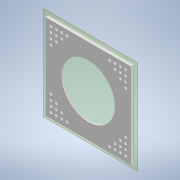
# Autodesk Inventor part: 60T-LocatorPlate
Saved by Autodesk Inventor 2020 (Build 240168000, 168)
## iProperties
Created: 2020-01-23
Part Number: 60T-LocatorPlate
Material: Generic
Document SubType Name: Modeling
Designer: srini
Density: 1 g/cm^3
Appearance: Default
Author: srini
Autodesk Inventor part; units mm, degrees
(part 1 of 2)
ref_plane "YZ Plane" through (0, 0, 0) normal (1, 0, 0) x (0, 1, 0)
ref_plane "XZ Plane" through (0, 0, 0) normal (0, 1, 0) x (-1, 0, 0)
ref_plane "XY Plane" through (0, 0, 0) normal (0, 0, 1) x (1, 0, 0)
sketch "Sketch1" plane through (0, 0, 0) normal (0, 0, 1) x (1, 0, 0)
  line L0 (-101.6, 101.6) -> (101.6, 101.6)
  line L1 (101.6, 101.6) -> (101.6, -101.6)
  line L2 (101.6, -101.6) -> (-101.6, -101.6)
  line L3 (-101.6, -101.6) -> (-101.6, 101.6)
  line L4 (-101.6, 101.6) -> (101.6, -101.6) construction
  line L5 (101.6, 101.6) -> (-101.6, -101.6) construction
  point P0 (0, 0)
  dimension "d0" = 203.2
  constraints: 12 end point, 2 midpoint, 2 parallel, 2 perpendicular, 1 horizontal
  measures "d0" distance of L0.start L0.end
extrude "Extrusion1" add sketch "Sketch1" along normal blind 3.175
ref_plane "Work Plane1" through (0, 0, -2.1465) normal (0, 0, -1) x (-1, 0, 0)
sketch "Sketch2" plane through (0, 0, -2.1465) normal (0, 0, -1) x (-1, 0, 0)
  circle A0 centre (0, 0) radius 14.3 construction
  circle A1 centre (20.6222, 11.9063) radius 2.1526 construction
  circle A2 centre (20.6222, -11.9062) radius 2.1526 construction
  circle A3 centre (0, -23.8125) radius 2.1526 construction
  circle A4 centre (-20.6222, -11.9063) radius 2.1526 construction
  circle A5 centre (-20.6222, 11.9062) radius 2.1526 construction
  circle A6 centre (0, 23.8125) radius 2.1526 construction
  arc A7 (-93.6337, -4.2799) -> (-93.5681, -5.531) centre (0, 0) ccw construction
  arc A8 (-92.0229, -3.2534) -> (-93.6337, -4.2799) centre (-90.7026, -7.1023) ccw construction
  line L0 (-92.0229, -3.2534) -> (-91.3043, -3.0069) construction
  arc A9 (-91.3043, -3.0069) -> (-89.552, -2.096) centre (-93.4636, 3.2878) ccw construction
  arc A10 (-89.552, -2.096) -> (-89.552, 2.096) centre (-91.0748, 0) ccw construction
  arc A11 (-89.552, 2.096) -> (-91.3043, 3.0069) centre (-93.4636, -3.2878) ccw construction
  line L1 (-91.3043, 3.0069) -> (-92.0229, 3.2534) construction
  arc A12 (-93.6337, 4.2799) -> (-92.0229, 3.2534) centre (-90.7026, 7.1023) ccw construction
  arc A13 (-93.5681, 5.531) -> (-93.6337, 4.2799) centre (0, 0) ccw construction
  arc A14 (-91.8588, 6.3834) -> (-93.5681, 5.531) centre (-90.9481, 2.4177) ccw construction
  line L2 (-91.8588, 6.3834) -> (-91.1184, 6.5535) construction
  arc A15 (-91.1184, 6.5535) -> (-89.2805, 7.2762) centre (-92.6079, 13.0394) ccw construction
  arc A16 (-89.2805, 7.2762) -> (-88.8423, 11.4453) centre (-90.5759, 9.5199) ccw construction
  arc A17 (-88.8423, 11.4453) -> (-90.4898, 12.5343) centre (-93.2953, 6.4998) ccw construction
  line L3 (-90.4898, 12.5343) -> (-91.1787, 12.8546) construction
  arc A18 (-92.6733, 14.0438) -> (-91.1787, 12.8546) centre (-89.4633, 16.5444) ccw construction
  arc A19 (-92.4774, 15.2812) -> (-92.6733, 14.0438) centre (0, 0) ccw construction
  arc A20 (-90.6884, 15.9503) -> (-92.4774, 15.2812) centre (-90.1972, 11.9111) ccw construction
  line L4 (-90.6884, 15.9503) -> (-89.9343, 16.042) construction
  arc A21 (-89.9343, 16.042) -> (-88.0308, 16.5687) centre (-90.7376, 22.6482) ccw construction
  arc A22 (-88.0308, 16.5687) -> (-87.1593, 20.6691) centre (-89.0846, 18.9355) ccw construction
  arc A23 (-87.1593, 20.6691) -> (-88.6839, 21.9244) centre (-92.1048, 16.2162) ccw construction
  line L5 (-88.6839, 21.9244) -> (-89.3355, 22.3149) construction
  arc A24 (-90.6977, 23.6539) -> (-89.3355, 22.3149) centre (-87.2439, 25.8052) ccw construction
  arc A25 (-90.3734, 24.864) -> (-90.6977, 23.6539) centre (0, 0) ccw construction
  arc A26 (-88.5243, 25.3425) -> (-90.3734, 24.864) centre (-88.458, 21.274) ccw construction
  line L6 (-88.5243, 25.3425) -> (-87.7647, 25.3548) construction
  arc A27 (-87.7647, 25.3548) -> (-85.8167, 25.6797) centre (-87.8731, 32.0088) ccw construction
  arc A28 (-85.8167, 25.6797) -> (-84.5213, 29.6665) centre (-86.6173, 28.1437) ccw construction
  arc A29 (-84.5213, 29.6665) -> (-85.9064, 31.0743) centre (-89.9051, 25.7549) ccw construction
  line L7 (-85.9064, 31.0743) -> (-86.5136, 31.5308) construction
  arc A30 (-87.7283, 33.0048) -> (-86.5136, 31.5308) centre (-84.0686, 34.7833) ccw construction
  arc A31 (-87.2794, 34.1744) -> (-87.7283, 33.0048) centre (0, 0) ccw construction
  arc A32 (-85.3904, 34.4569) -> (-87.2794, 34.1744) centre (-85.7497, 30.4038) ccw construction
  line L8 (-85.3904, 34.4569) -> (-84.6337, 34.3899) construction
  arc A33 (-84.6337, 34.3899) -> (-82.6623, 34.5093) centre (-84.0459, 41.0187) ccw construction
  arc A34 (-82.6623, 34.5093) -> (-80.9573, 38.3389) centre (-83.201, 37.0435) ccw construction
  arc A35 (-80.9573, 38.3389) -> (-82.1876, 39.8837) centre (-86.7205, 35.0115) ccw construction
  line L9 (-82.1876, 39.8837) -> (-82.7438, 40.4012) construction
  arc A36 (-83.7978, 41.9941) -> (-82.7438, 40.4012) centre (-79.9722, 43.3803) ccw construction
  arc A37 (-83.2291, 43.1103) -> (-83.7978, 41.9941) centre (0, 0) ccw construction
  arc A38 (-81.3208, 43.1939) -> (-83.2291, 43.1103) centre (-82.1019, 39.2006) ccw construction
  line L10 (-81.3208, 43.1939) -> (-80.5753, 43.0481) construction
  arc A39 (-80.5753, 43.0481) -> (-78.6023, 42.9608) centre (-79.2979, 49.5791) ccw construction
  arc A40 (-78.6023, 42.9608) -> (-76.5063, 46.5912) centre (-78.8731, 45.5374) ccw construction
  arc A41 (-76.5063, 46.5912) -> (-77.5684, 48.2562) centre (-82.5858, 43.8844) ccw construction
  line L11 (-77.5684, 48.2562) -> (-78.0675, 48.829) construction
  arc A42 (-78.9492, 50.5233) -> (-78.0675, 48.829) centre (-74.9996, 51.502) ccw construction
  arc A43 (-78.2669, 51.574) -> (-78.9492, 50.5233) centre (0, 0) ccw construction
  arc A44 (-76.3604, 51.4576) -> (-78.2669, 51.574) centre (-77.5546, 47.5678) ccw construction
  line L12 (-76.3604, 51.4576) -> (-75.6342, 51.2347) construction
  arc A45 (-75.6342, 51.2347) -> (-73.6811, 50.9416) centre (-73.6811, 57.5964) ccw construction
  arc A46 (-73.6811, 50.9416) -> (-71.2171, 54.333) centre (-73.6811, 53.5324) ccw construction
  arc A47 (-71.2171, 54.333) -> (-72.0993, 56.1) centre (-77.5462, 52.2766) ccw construction
  line L13 (-72.0993, 56.1) -> (-72.5358, 56.7217) construction
  arc A48 (-73.2356, 58.499) -> (-72.5358, 56.7217) centre (-69.2054, 59.0595) ccw construction
  arc A49 (-72.4472, 59.4726) -> (-73.2356, 58.499) centre (0, 0) ccw construction
  arc A50 (-70.5633, 59.1576) -> (-72.4472, 59.4726) centre (-72.1575, 55.4139) ccw construction
  line L14 (-70.5633, 59.1576) -> (-69.8643, 58.8599) construction
  arc A51 (-69.8643, 58.8599) -> (-67.9526, 58.3643) centre (-67.257, 64.9827) ccw construction
  arc A52 (-67.9526, 58.3643) -> (-65.1476, 61.4796) centre (-67.6818, 60.9409) ccw construction
  arc A53 (-65.1476, 61.4796) -> (-65.8403, 63.3291) centre (-71.657, 60.096) ccw construction
  line L15 (-65.8403, 63.3291) -> (-66.2094, 63.9931) construction
  arc A54 (-66.7196, 65.8337) -> (-66.2094, 63.9931) centre (-62.6528, 65.9699) ccw construction
  arc A55 (-65.8337, 66.7196) -> (-66.7196, 65.8337) centre (0, 0) ccw construction
  arc A56 (-63.9931, 66.2094) -> (-65.8337, 66.7196) centre (-65.9699, 62.6528) ccw construction
  line L16 (-63.9931, 66.2094) -> (-63.3291, 65.8403) construction
  arc A57 (-63.3291, 65.8403) -> (-61.4796, 65.1476) centre (-60.096, 71.657) ccw construction
  arc A58 (-61.4796, 65.1476) -> (-58.3643, 67.9526) centre (-60.941, 67.6818) ccw construction
  arc A59 (-58.3643, 67.9526) -> (-58.8599, 69.8643) centre (-64.9827, 67.257) ccw construction
  line L17 (-58.8599, 69.8643) -> (-59.1576, 70.5633) construction
  arc A60 (-59.4726, 72.4472) -> (-59.1576, 70.5633) centre (-55.4139, 72.1575) ccw construction
  arc A61 (-58.499, 73.2356) -> (-59.4726, 72.4472) centre (0, 0) ccw construction
  arc A62 (-56.7217, 72.5358) -> (-58.499, 73.2356) centre (-59.0595, 69.2053) ccw construction
  line L18 (-56.7217, 72.5358) -> (-56.1, 72.0993) construction
  arc A63 (-56.1, 72.0993) -> (-54.333, 71.2171) centre (-52.2766, 77.5462) ccw construction
  arc A64 (-54.333, 71.2171) -> (-50.9416, 73.6811) centre (-53.5324, 73.6811) ccw construction
  arc A65 (-50.9416, 73.6811) -> (-51.2347, 75.6341) centre (-57.5964, 73.6811) ccw construction
  line L19 (-51.2347, 75.6341) -> (-51.4576, 76.3604) construction
  arc A66 (-51.574, 78.2669) -> (-51.4576, 76.3604) centre (-47.5678, 77.5545) ccw construction
  arc A67 (-50.5233, 78.9492) -> (-51.574, 78.2669) centre (0, 0) ccw construction
  arc A68 (-48.829, 78.0674) -> (-50.5233, 78.9492) centre (-51.502, 74.9996) ccw construction
  line L20 (-48.829, 78.0674) -> (-48.2562, 77.5684) construction
  arc A69 (-48.2562, 77.5684) -> (-46.5912, 76.5063) centre (-43.8844, 82.5858) ccw construction
  arc A70 (-46.5912, 76.5063) -> (-42.9608, 78.6023) centre (-45.5374, 78.8731) ccw construction
  arc A71 (-42.9608, 78.6023) -> (-43.0481, 80.5753) centre (-49.5792, 79.2979) ccw construction
  line L21 (-43.0481, 80.5753) -> (-43.1939, 81.3208) construction
  arc A72 (-43.1103, 83.2291) -> (-43.1939, 81.3208) centre (-39.2006, 82.1019) ccw construction
  arc A73 (-41.9941, 83.7978) -> (-43.1103, 83.2291) centre (0, 0) ccw construction
  arc A74 (-40.4012, 82.7438) -> (-41.9941, 83.7978) centre (-43.3803, 79.9722) ccw construction
  line L22 (-40.4012, 82.7438) -> (-39.8838, 82.1876) construction
  arc A75 (-39.8838, 82.1876) -> (-38.3389, 80.9573) centre (-35.0115, 86.7205) ccw construction
  arc A76 (-38.3389, 80.9573) -> (-34.5093, 82.6623) centre (-37.0435, 83.201) ccw construction
  arc A77 (-34.5093, 82.6623) -> (-34.3899, 84.6336) centre (-41.0187, 84.0459) ccw construction
  line L23 (-34.3899, 84.6336) -> (-34.457, 85.3904) construction
  arc A78 (-34.1744, 87.2794) -> (-34.457, 85.3904) centre (-30.4038, 85.7497) ccw construction
  arc A79 (-33.0048, 87.7283) -> (-34.1744, 87.2794) centre (0, 0) ccw construction
  arc A80 (-31.5308, 86.5136) -> (-33.0048, 87.7283) centre (-34.7833, 84.0686) ccw construction
  line L24 (-31.5308, 86.5136) -> (-31.0743, 85.9064) construction
  arc A81 (-31.0743, 85.9064) -> (-29.6665, 84.5213) centre (-25.7549, 89.9051) ccw construction
  arc A82 (-29.6665, 84.5213) -> (-25.6797, 85.8167) centre (-28.1437, 86.6173) ccw construction
  arc A83 (-25.6797, 85.8167) -> (-25.3548, 87.7647) centre (-32.0088, 87.8731) ccw construction
  line L25 (-25.3548, 87.7647) -> (-25.3425, 88.5243) construction
  arc A84 (-24.864, 90.3734) -> (-25.3425, 88.5243) centre (-21.274, 88.458) ccw construction
  arc A85 (-23.6539, 90.6977) -> (-24.864, 90.3734) centre (0, 0) ccw construction
  arc A86 (-22.3149, 89.3355) -> (-23.6539, 90.6977) centre (-25.8052, 87.2439) ccw construction
  line L26 (-22.3149, 89.3355) -> (-21.9244, 88.6839) construction
  arc A87 (-21.9244, 88.6839) -> (-20.6691, 87.1593) centre (-16.2162, 92.1048) ccw construction
  arc A88 (-20.6691, 87.1593) -> (-16.5687, 88.0308) centre (-18.9355, 89.0846) ccw construction
  arc A89 (-16.5687, 88.0308) -> (-16.042, 89.9343) centre (-22.6482, 90.7376) ccw construction
  line L27 (-16.042, 89.9343) -> (-15.9503, 90.6884) construction
  arc A90 (-15.2812, 92.4774) -> (-15.9503, 90.6884) centre (-11.9111, 90.1972) ccw construction
  arc A91 (-14.0438, 92.6733) -> (-15.2812, 92.4774) centre (0, 0) ccw construction
  arc A92 (-12.8546, 91.1787) -> (-14.0438, 92.6733) centre (-16.5444, 89.4633) ccw construction
  line L28 (-12.8546, 91.1787) -> (-12.5343, 90.4898) construction
  arc A93 (-12.5343, 90.4898) -> (-11.4453, 88.8423) centre (-6.4998, 93.2952) ccw construction
  arc A94 (-11.4453, 88.8423) -> (-7.2762, 89.2805) centre (-9.5199, 90.5759) ccw construction
  arc A95 (-7.2762, 89.2805) -> (-6.5535, 91.1184) centre (-13.0394, 92.6079) ccw construction
  line L29 (-6.5535, 91.1184) -> (-6.3834, 91.8588) construction
  arc A96 (-5.531, 93.5681) -> (-6.3834, 91.8588) centre (-2.4177, 90.9481) ccw construction
  arc A97 (-4.2799, 93.6336) -> (-5.531, 93.5681) centre (0, 0) ccw construction
  arc A98 (-3.2534, 92.0229) -> (-4.2799, 93.6336) centre (-7.1023, 90.7026) ccw construction
  line L30 (-3.2534, 92.0229) -> (-3.0069, 91.3043) construction
  arc A99 (-3.0069, 91.3043) -> (-2.096, 89.552) centre (3.2878, 93.4636) ccw construction
  arc A100 (-2.096, 89.552) -> (2.096, 89.552) centre (0, 91.0748) ccw construction
  arc A101 (2.096, 89.552) -> (3.0069, 91.3043) centre (-3.2878, 93.4636) ccw construction
  line L31 (3.0069, 91.3043) -> (3.2534, 92.0229) construction
  arc A102 (4.2799, 93.6336) -> (3.2534, 92.0229) centre (7.1022, 90.7026) ccw construction
  arc A103 (5.5309, 93.5681) -> (4.2799, 93.6336) centre (0, 0) ccw construction
  arc A104 (6.3834, 91.8588) -> (5.5309, 93.5681) centre (2.4177, 90.9481) ccw construction
  line L32 (6.3834, 91.8588) -> (6.5535, 91.1184) construction
  arc A105 (6.5535, 91.1184) -> (7.2762, 89.2805) centre (13.0394, 92.6079) ccw construction
  arc A106 (7.2762, 89.2805) -> (11.4452, 88.8423) centre (9.5199, 90.5759) ccw construction
  arc A107 (11.4452, 88.8423) -> (12.5343, 90.4898) centre (6.4998, 93.2952) ccw construction
  line L33 (12.5343, 90.4898) -> (12.8546, 91.1787) construction
  arc A108 (14.0438, 92.6733) -> (12.8546, 91.1787) centre (16.5443, 89.4633) ccw construction
  arc A109 (15.2812, 92.4774) -> (14.0438, 92.6733) centre (0, 0) ccw construction
  arc A110 (15.9503, 90.6884) -> (15.2812, 92.4774) centre (11.9111, 90.1972) ccw construction
  line L34 (15.9503, 90.6884) -> (16.042, 89.9343) construction
  arc A111 (16.042, 89.9343) -> (16.5687, 88.0308) centre (22.6482, 90.7376) ccw construction
  arc A112 (16.5687, 88.0308) -> (20.6691, 87.1593) centre (18.9355, 89.0846) ccw construction
  arc A113 (20.6691, 87.1593) -> (21.9244, 88.6839) centre (16.2162, 92.1048) ccw construction
  line L35 (21.9244, 88.6839) -> (22.3149, 89.3355) construction
  arc A114 (23.6539, 90.6977) -> (22.3149, 89.3355) centre (25.8052, 87.2439) ccw construction
  arc A115 (24.864, 90.3734) -> (23.6539, 90.6977) centre (0, 0) ccw construction
  arc A116 (25.3425, 88.5243) -> (24.864, 90.3734) centre (21.274, 88.458) ccw construction
  line L36 (25.3425, 88.5243) -> (25.3548, 87.7647) construction
  arc A117 (25.3548, 87.7647) -> (25.6797, 85.8167) centre (32.0088, 87.8731) ccw construction
  arc A118 (25.6797, 85.8167) -> (29.6665, 84.5213) centre (28.1437, 86.6173) ccw construction
  arc A119 (29.6665, 84.5213) -> (31.0743, 85.9064) centre (25.7549, 89.9051) ccw construction
  line L37 (31.0743, 85.9064) -> (31.5308, 86.5136) construction
  arc A120 (33.0048, 87.7283) -> (31.5308, 86.5136) centre (34.7833, 84.0686) ccw construction
  arc A121 (34.1744, 87.2794) -> (33.0048, 87.7283) centre (0, 0) ccw construction
  arc A122 (34.4569, 85.3903) -> (34.1744, 87.2794) centre (30.4038, 85.7497) ccw construction
  line L38 (34.4569, 85.3903) -> (34.3899, 84.6337) construction
  arc A123 (34.3899, 84.6337) -> (34.5093, 82.6623) centre (41.0187, 84.0459) ccw construction
  arc A124 (34.5093, 82.6623) -> (38.3389, 80.9573) centre (37.0435, 83.201) ccw construction
  arc A125 (38.3389, 80.9573) -> (39.8837, 82.1876) centre (35.0115, 86.7205) ccw construction
  line L39 (39.8837, 82.1876) -> (40.4012, 82.7438) construction
  arc A126 (41.9941, 83.7978) -> (40.4012, 82.7438) centre (43.3803, 79.9722) ccw construction
  arc A127 (43.1103, 83.2291) -> (41.9941, 83.7978) centre (0, 0) ccw construction
  arc A128 (43.1939, 81.3208) -> (43.1103, 83.2291) centre (39.2006, 82.1019) ccw construction
  line L40 (43.1939, 81.3208) -> (43.0481, 80.5753) construction
  arc A129 (43.0481, 80.5753) -> (42.9608, 78.6023) centre (49.5791, 79.2979) ccw construction
  arc A130 (42.9608, 78.6023) -> (46.5912, 76.5063) centre (45.5374, 78.8731) ccw construction
  arc A131 (46.5912, 76.5063) -> (48.2562, 77.5684) centre (43.8844, 82.5858) ccw construction
  line L41 (48.2562, 77.5684) -> (48.829, 78.0674) construction
  arc A132 (50.5233, 78.9492) -> (48.829, 78.0674) centre (51.502, 74.9996) ccw construction
  arc A133 (51.574, 78.2669) -> (50.5233, 78.9492) centre (0, 0) ccw construction
  arc A134 (51.4576, 76.3604) -> (51.574, 78.2669) centre (47.5678, 77.5545) ccw construction
  line L42 (51.4576, 76.3604) -> (51.2347, 75.6342) construction
  arc A135 (51.2347, 75.6342) -> (50.9416, 73.6811) centre (57.5964, 73.6811) ccw construction
  arc A136 (50.9416, 73.6811) -> (54.333, 71.2171) centre (53.5324, 73.6811) ccw construction
  arc A137 (54.333, 71.2171) -> (56.1, 72.0993) centre (52.2766, 77.5462) ccw construction
  line L43 (56.1, 72.0993) -> (56.7217, 72.5358) construction
  arc A138 (58.499, 73.2356) -> (56.7217, 72.5358) centre (59.0595, 69.2053) ccw construction
  arc A139 (59.4726, 72.4472) -> (58.499, 73.2356) centre (0, 0) ccw construction
  arc A140 (59.1576, 70.5633) -> (59.4726, 72.4472) centre (55.4139, 72.1575) ccw construction
  line L44 (59.1576, 70.5633) -> (58.8599, 69.8643) construction
  arc A141 (58.8599, 69.8643) -> (58.3643, 67.9526) centre (64.9827, 67.257) ccw construction
  arc A142 (58.3643, 67.9526) -> (61.4796, 65.1476) centre (60.9409, 67.6818) ccw construction
  arc A143 (61.4796, 65.1476) -> (63.3291, 65.8403) centre (60.096, 71.657) ccw construction
  line L45 (63.3291, 65.8403) -> (63.9931, 66.2094) construction
  arc A144 (65.8337, 66.7196) -> (63.9931, 66.2094) centre (65.9699, 62.6528) ccw construction
  arc A145 (66.7196, 65.8337) -> (65.8337, 66.7196) centre (0, 0) ccw construction
  arc A146 (66.2094, 63.9931) -> (66.7196, 65.8337) centre (62.6528, 65.9699) ccw construction
  line L46 (66.2094, 63.9931) -> (65.8403, 63.3291) construction
  arc A147 (65.8403, 63.3291) -> (65.1476, 61.4796) centre (71.657, 60.096) ccw construction
  arc A148 (65.1476, 61.4796) -> (67.9526, 58.3643) centre (67.6818, 60.9409) ccw construction
  arc A149 (67.9526, 58.3643) -> (69.8643, 58.8599) centre (67.257, 64.9827) ccw construction
  line L47 (69.8643, 58.8599) -> (70.5633, 59.1576) construction
  arc A150 (72.4472, 59.4726) -> (70.5633, 59.1576) centre (72.1575, 55.4139) ccw construction
  arc A151 (73.2356, 58.499) -> (72.4472, 59.4726) centre (0, 0) ccw construction
  arc A152 (72.5358, 56.7217) -> (73.2356, 58.499) centre (69.2053, 59.0595) ccw construction
  line L48 (72.5358, 56.7217) -> (72.0993, 56.1) construction
  arc A153 (72.0993, 56.1) -> (71.2171, 54.333) centre (77.5462, 52.2766) ccw construction
  arc A154 (71.2171, 54.333) -> (73.6811, 50.9416) centre (73.6811, 53.5324) ccw construction
  arc A155 (73.6811, 50.9416) -> (75.6341, 51.2347) centre (73.6811, 57.5964) ccw construction
  line L49 (75.6341, 51.2347) -> (76.3604, 51.4576) construction
  arc A156 (78.2669, 51.574) -> (76.3604, 51.4576) centre (77.5545, 47.5678) ccw construction
  arc A157 (78.9492, 50.5233) -> (78.2669, 51.574) centre (0, 0) ccw construction
  arc A158 (78.0674, 48.829) -> (78.9492, 50.5233) centre (74.9996, 51.502) ccw construction
  line L50 (78.0674, 48.829) -> (77.5684, 48.2562) construction
  arc A159 (77.5684, 48.2562) -> (76.5063, 46.5912) centre (82.5858, 43.8844) ccw construction
  arc A160 (76.5063, 46.5912) -> (78.6023, 42.9608) centre (78.8731, 45.5374) ccw construction
  arc A161 (78.6023, 42.9608) -> (80.5753, 43.0481) centre (79.2979, 49.5791) ccw construction
  line L51 (80.5753, 43.0481) -> (81.3208, 43.1939) construction
  arc A162 (83.229, 43.1103) -> (81.3208, 43.1939) centre (82.1019, 39.2006) ccw construction
  arc A163 (83.7978, 41.9941) -> (83.229, 43.1103) centre (0, 0) ccw construction
  arc A164 (82.7438, 40.4012) -> (83.7978, 41.9941) centre (79.9722, 43.3803) ccw construction
  line L52 (82.7438, 40.4012) -> (82.1876, 39.8838) construction
  arc A165 (82.1876, 39.8838) -> (80.9573, 38.3389) centre (86.7205, 35.0115) ccw construction
  arc A166 (80.9573, 38.3389) -> (82.6623, 34.5093) centre (83.201, 37.0435) ccw construction
  arc A167 (82.6623, 34.5093) -> (84.6336, 34.3899) centre (84.0459, 41.0187) ccw construction
  line L53 (84.6336, 34.3899) -> (85.3903, 34.4569) construction
  arc A168 (87.2794, 34.1744) -> (85.3903, 34.4569) centre (85.7497, 30.4038) ccw construction
  arc A169 (87.7283, 33.0048) -> (87.2794, 34.1744) centre (0, 0) ccw construction
  arc A170 (86.5136, 31.5308) -> (87.7283, 33.0048) centre (84.0686, 34.7833) ccw construction
  line L54 (86.5136, 31.5308) -> (85.9064, 31.0743) construction
  arc A171 (85.9064, 31.0743) -> (84.5213, 29.6665) centre (89.9051, 25.7549) ccw construction
  arc A172 (84.5213, 29.6665) -> (85.8167, 25.6797) centre (86.6173, 28.1437) ccw construction
  arc A173 (85.8167, 25.6797) -> (87.7647, 25.3548) centre (87.8731, 32.0088) ccw construction
  line L55 (87.7647, 25.3548) -> (88.5243, 25.3425) construction
  arc A174 (90.3734, 24.864) -> (88.5243, 25.3425) centre (88.458, 21.274) ccw construction
  arc A175 (90.6977, 23.6539) -> (90.3734, 24.864) centre (0, 0) ccw construction
  arc A176 (89.3355, 22.3149) -> (90.6977, 23.6539) centre (87.2439, 25.8052) ccw construction
  line L56 (89.3355, 22.3149) -> (88.6839, 21.9244) construction
  arc A177 (88.6839, 21.9244) -> (87.1593, 20.6691) centre (92.1048, 16.2162) ccw construction
  arc A178 (87.1593, 20.6691) -> (88.0308, 16.5687) centre (89.0846, 18.9355) ccw construction
  arc A179 (88.0308, 16.5687) -> (89.9342, 16.042) centre (90.7376, 22.6482) ccw construction
  line L57 (89.9342, 16.042) -> (90.6884, 15.9503) construction
  arc A180 (92.4774, 15.2812) -> (90.6884, 15.9503) centre (90.1972, 11.9111) ccw construction
  arc A181 (92.6733, 14.0438) -> (92.4774, 15.2812) centre (0, 0) ccw construction
  arc A182 (91.1787, 12.8546) -> (92.6733, 14.0438) centre (89.4633, 16.5443) ccw construction
  line L58 (91.1787, 12.8546) -> (90.4898, 12.5343) construction
  arc A183 (90.4898, 12.5343) -> (88.8423, 11.4452) centre (93.2952, 6.4998) ccw construction
  arc A184 (88.8423, 11.4452) -> (89.2805, 7.2762) centre (90.5759, 9.5199) ccw construction
  arc A185 (89.2805, 7.2762) -> (91.1184, 6.5535) centre (92.6079, 13.0394) ccw construction
  line L59 (91.1184, 6.5535) -> (91.8588, 6.3834) construction
  arc A186 (93.5681, 5.5309) -> (91.8588, 6.3834) centre (90.9481, 2.4177) ccw construction
  arc A187 (93.6336, 4.2799) -> (93.5681, 5.5309) centre (0, 0) ccw construction
  arc A188 (92.0229, 3.2534) -> (93.6336, 4.2799) centre (90.7026, 7.1022) ccw construction
  line L60 (92.0229, 3.2534) -> (91.3043, 3.0069) construction
  arc A189 (91.3043, 3.0069) -> (89.552, 2.096) centre (93.4636, -3.2878) ccw construction
  arc A190 (89.552, 2.096) -> (89.552, -2.096) centre (91.0748, 0) ccw construction
  arc A191 (89.552, -2.096) -> (91.3043, -3.0069) centre (93.4636, 3.2878) ccw construction
  line L61 (91.3043, -3.0069) -> (92.0229, -3.2534) construction
  arc A192 (93.6336, -4.2799) -> (92.0229, -3.2534) centre (90.7026, -7.1023) ccw construction
  arc A193 (93.5681, -5.531) -> (93.6336, -4.2799) centre (0, 0) ccw construction
  arc A194 (91.8588, -6.3834) -> (93.5681, -5.531) centre (90.9481, -2.4177) ccw construction
  line L62 (91.8588, -6.3834) -> (91.1184, -6.5535) construction
  arc A195 (91.1184, -6.5535) -> (89.2805, -7.2762) centre (92.6079, -13.0394) ccw construction
  arc A196 (89.2805, -7.2762) -> (88.8423, -11.4453) centre (90.5759, -9.5199) ccw construction
  arc A197 (88.8423, -11.4453) -> (90.4898, -12.5343) centre (93.2952, -6.4998) ccw construction
  line L63 (90.4898, -12.5343) -> (91.1787, -12.8546) construction
  arc A198 (92.6733, -14.0438) -> (91.1787, -12.8546) centre (89.4633, -16.5444) ccw construction
  arc A199 (92.4774, -15.2812) -> (92.6733, -14.0438) centre (0, 0) ccw construction
  arc A200 (90.6884, -15.9503) -> (92.4774, -15.2812) centre (90.1972, -11.9111) ccw construction
  line L64 (90.6884, -15.9503) -> (89.9343, -16.042) construction
  arc A201 (89.9343, -16.042) -> (88.0308, -16.5687) centre (90.7376, -22.6482) ccw construction
  arc A202 (88.0308, -16.5687) -> (87.1593, -20.6691) centre (89.0846, -18.9355) ccw construction
  arc A203 (87.1593, -20.6691) -> (88.6839, -21.9244) centre (92.1048, -16.2162) ccw construction
  line L65 (88.6839, -21.9244) -> (89.3355, -22.3149) construction
  arc A204 (90.6977, -23.6539) -> (89.3355, -22.3149) centre (87.2439, -25.8052) ccw construction
  arc A205 (90.3734, -24.864) -> (90.6977, -23.6539) centre (0, 0) ccw construction
  arc A206 (88.5243, -25.3425) -> (90.3734, -24.864) centre (88.458, -21.274) ccw construction
  line L66 (88.5243, -25.3425) -> (87.7647, -25.3548) construction
  arc A207 (87.7647, -25.3548) -> (85.8167, -25.6797) centre (87.8731, -32.0088) ccw construction
  arc A208 (85.8167, -25.6797) -> (84.5213, -29.6665) centre (86.6173, -28.1437) ccw construction
  arc A209 (84.5213, -29.6665) -> (85.9064, -31.0743) centre (89.9051, -25.7549) ccw construction
  line L67 (85.9064, -31.0743) -> (86.5136, -31.5308) construction
  arc A210 (87.7283, -33.0048) -> (86.5136, -31.5308) centre (84.0686, -34.7833) ccw construction
  arc A211 (87.2794, -34.1744) -> (87.7283, -33.0048) centre (0, 0) ccw construction
  arc A212 (85.3903, -34.457) -> (87.2794, -34.1744) centre (85.7497, -30.4038) ccw construction
  line L68 (85.3903, -34.457) -> (84.6337, -34.3899) construction
  arc A213 (84.6337, -34.3899) -> (82.6623, -34.5093) centre (84.0459, -41.0187) ccw construction
  arc A214 (82.6623, -34.5093) -> (80.9573, -38.3389) centre (83.201, -37.0435) ccw construction
  arc A215 (80.9573, -38.3389) -> (82.1876, -39.8838) centre (86.7205, -35.0115) ccw construction
  line L69 (82.1876, -39.8838) -> (82.7438, -40.4012) construction
  arc A216 (83.7978, -41.9941) -> (82.7438, -40.4012) centre (79.9722, -43.3803) ccw construction
  arc A217 (83.229, -43.1103) -> (83.7978, -41.9941) centre (0, 0) ccw construction
  arc A218 (81.3208, -43.1939) -> (83.229, -43.1103) centre (82.1019, -39.2006) ccw construction
  line L70 (81.3208, -43.1939) -> (80.5753, -43.0481) construction
  arc A219 (80.5753, -43.0481) -> (78.6023, -42.9608) centre (79.2979, -49.5791) ccw construction
  arc A220 (78.6023, -42.9608) -> (76.5063, -46.5912) centre (78.8731, -45.5374) ccw construction
  arc A221 (76.5063, -46.5912) -> (77.5684, -48.2562) centre (82.5857, -43.8844) ccw construction
  line L71 (77.5684, -48.2562) -> (78.0674, -48.829) construction
  arc A222 (78.9492, -50.5233) -> (78.0674, -48.829) centre (74.9996, -51.502) ccw construction
  arc A223 (78.2669, -51.574) -> (78.9492, -50.5233) centre (0, 0) ccw construction
  arc A224 (76.3604, -51.4576) -> (78.2669, -51.574) centre (77.5545, -47.5678) ccw construction
  line L72 (76.3604, -51.4576) -> (75.6341, -51.2347) construction
  arc A225 (75.6341, -51.2347) -> (73.6811, -50.9416) centre (73.6811, -57.5964) ccw construction
  arc A226 (73.6811, -50.9416) -> (71.2171, -54.333) centre (73.6811, -53.5324) ccw construction
  arc A227 (71.2171, -54.333) -> (72.0993, -56.1) centre (77.5462, -52.2766) ccw construction
  line L73 (72.0993, -56.1) -> (72.5358, -56.7217) construction
  arc A228 (73.2356, -58.499) -> (72.5358, -56.7217) centre (69.2053, -59.0595) ccw construction
  arc A229 (72.4471, -59.4726) -> (73.2356, -58.499) centre (0, 0) ccw construction
  arc A230 (70.5633, -59.1576) -> (72.4471, -59.4726) centre (72.1575, -55.4139) ccw construction
  line L74 (70.5633, -59.1576) -> (69.8643, -58.8599) construction
  arc A231 (69.8643, -58.8599) -> (67.9526, -58.3643) centre (67.257, -64.9827) ccw construction
  arc A232 (67.9526, -58.3643) -> (65.1476, -61.4796) centre (67.6818, -60.941) ccw construction
  arc A233 (65.1476, -61.4796) -> (65.8403, -63.3291) centre (71.657, -60.096) ccw construction
  line L75 (65.8403, -63.3291) -> (66.2094, -63.9931) construction
  arc A234 (66.7196, -65.8337) -> (66.2094, -63.9931) centre (62.6528, -65.9699) ccw construction
  arc A235 (65.8337, -66.7196) -> (66.7196, -65.8337) centre (0, 0) ccw construction
  arc A236 (63.9931, -66.2094) -> (65.8337, -66.7196) centre (65.9699, -62.6528) ccw construction
  line L76 (63.9931, -66.2094) -> (63.3291, -65.8403) construction
  arc A237 (63.3291, -65.8403) -> (61.4796, -65.1476) centre (60.096, -71.657) ccw construction
  arc A238 (61.4796, -65.1476) -> (58.3643, -67.9526) centre (60.9409, -67.6818) ccw construction
  arc A239 (58.3643, -67.9526) -> (58.8599, -69.8643) centre (64.9827, -67.257) ccw construction
  line L77 (58.8599, -69.8643) -> (59.1576, -70.5633) construction
  arc A240 (59.4726, -72.4472) -> (59.1576, -70.5633) centre (55.4139, -72.1575) ccw construction
  arc A241 (58.499, -73.2356) -> (59.4726, -72.4472) centre (0, 0) ccw construction
  arc A242 (56.7217, -72.5358) -> (58.499, -73.2356) centre (59.0595, -69.2054) ccw construction
  line L78 (56.7217, -72.5358) -> (56.1, -72.0993) construction
  arc A243 (56.1, -72.0993) -> (54.333, -71.2171) centre (52.2766, -77.5462) ccw construction
  arc A244 (54.333, -71.2171) -> (50.9416, -73.6811) centre (53.5324, -73.6811) ccw construction
  arc A245 (50.9416, -73.6811) -> (51.2347, -75.6341) centre (57.5964, -73.6811) ccw construction
  line L79 (51.2347, -75.6341) -> (51.4576, -76.3604) construction
  arc A246 (51.574, -78.2669) -> (51.4576, -76.3604) centre (47.5678, -77.5546) ccw construction
  arc A247 (50.5233, -78.9492) -> (51.574, -78.2669) centre (0, 0) ccw construction
  arc A248 (48.8289, -78.0674) -> (50.5233, -78.9492) centre (51.502, -74.9996) ccw construction
  line L80 (48.8289, -78.0674) -> (48.2562, -77.5684) construction
  arc A249 (48.2562, -77.5684) -> (46.5912, -76.5063) centre (43.8844, -82.5858) ccw construction
  arc A250 (46.5912, -76.5063) -> (42.9608, -78.6023) centre (45.5374, -78.8731) ccw construction
  arc A251 (42.9608, -78.6023) -> (43.0481, -80.5753) centre (49.5791, -79.2979) ccw construction
  line L81 (43.0481, -80.5753) -> (43.1939, -81.3208) construction
  arc A252 (43.1103, -83.2291) -> (43.1939, -81.3208) centre (39.2006, -82.1019) ccw construction
  arc A253 (41.9941, -83.7978) -> (43.1103, -83.2291) centre (0, 0) ccw construction
  arc A254 (40.4012, -82.7438) -> (41.9941, -83.7978) centre (43.3803, -79.9722) ccw construction
  line L82 (40.4012, -82.7438) -> (39.8837, -82.1876) construction
  arc A255 (39.8837, -82.1876) -> (38.3389, -80.9573) centre (35.0115, -86.7205) ccw construction
  arc A256 (38.3389, -80.9573) -> (34.5093, -82.6623) centre (37.0435, -83.201) ccw construction
  arc A257 (34.5093, -82.6623) -> (34.3899, -84.6336) centre (41.0187, -84.0459) ccw construction
  line L83 (34.3899, -84.6336) -> (34.4569, -85.3904) construction
  arc A258 (34.1744, -87.2794) -> (34.4569, -85.3904) centre (30.4038, -85.7497) ccw construction
  arc A259 (33.0048, -87.7283) -> (34.1744, -87.2794) centre (0, 0) ccw construction
  arc A260 (31.5308, -86.5136) -> (33.0048, -87.7283) centre (34.7833, -84.0686) ccw construction
  line L84 (31.5308, -86.5136) -> (31.0743, -85.9064) construction
  arc A261 (31.0743, -85.9064) -> (29.6665, -84.5213) centre (25.7549, -89.9051) ccw construction
  arc A262 (29.6665, -84.5213) -> (25.6797, -85.8167) centre (28.1437, -86.6173) ccw construction
  arc A263 (25.6797, -85.8167) -> (25.3548, -87.7647) centre (32.0088, -87.8731) ccw construction
  line L85 (25.3548, -87.7647) -> (25.3425, -88.5243) construction
  arc A264 (24.864, -90.3734) -> (25.3425, -88.5243) centre (21.274, -88.458) ccw construction
  arc A265 (23.6539, -90.6977) -> (24.864, -90.3734) centre (0, 0) ccw construction
  arc A266 (22.3149, -89.3355) -> (23.6539, -90.6977) centre (25.8052, -87.2439) ccw construction
  line L86 (22.3149, -89.3355) -> (21.9244, -88.6839) construction
  arc A267 (21.9244, -88.6839) -> (20.6691, -87.1593) centre (16.2162, -92.1048) ccw construction
  arc A268 (20.6691, -87.1593) -> (16.5687, -88.0308) centre (18.9355, -89.0846) ccw construction
  arc A269 (16.5687, -88.0308) -> (16.042, -89.9343) centre (22.6482, -90.7376) ccw construction
  line L87 (16.042, -89.9343) -> (15.9503, -90.6884) construction
  arc A270 (15.2812, -92.4774) -> (15.9503, -90.6884) centre (11.9111, -90.1972) ccw construction
  arc A271 (14.0438, -92.6733) -> (15.2812, -92.4774) centre (0, 0) ccw construction
  arc A272 (12.8546, -91.1787) -> (14.0438, -92.6733) centre (16.5443, -89.4633) ccw construction
  line L88 (12.8546, -91.1787) -> (12.5343, -90.4898) construction
  arc A273 (12.5343, -90.4898) -> (11.4452, -88.8423) centre (6.4998, -93.2952) ccw construction
  arc A274 (11.4452, -88.8423) -> (7.2762, -89.2805) centre (9.5199, -90.5759) ccw construction
  arc A275 (7.2762, -89.2805) -> (6.5535, -91.1184) centre (13.0394, -92.6079) ccw construction
  line L89 (6.5535, -91.1184) -> (6.3834, -91.8588) construction
  arc A276 (5.5309, -93.5681) -> (6.3834, -91.8588) centre (2.4177, -90.9481) ccw construction
  arc A277 (4.2799, -93.6336) -> (5.5309, -93.5681) centre (0, 0) ccw construction
  arc A278 (3.2534, -92.0229) -> (4.2799, -93.6336) centre (7.1022, -90.7026) ccw construction
  line L90 (3.2534, -92.0229) -> (3.0069, -91.3043) construction
  arc A279 (3.0069, -91.3043) -> (2.096, -89.552) centre (-3.2879, -93.4636) ccw construction
  arc A280 (2.096, -89.552) -> (-2.096, -89.552) centre (0, -91.0748) ccw construction
  arc A281 (-2.096, -89.552) -> (-3.0069, -91.3043) centre (3.2878, -93.4636) ccw construction
  line L91 (-3.0069, -91.3043) -> (-3.2534, -92.0229) construction
  arc A282 (-4.2799, -93.6336) -> (-3.2534, -92.0229) centre (-7.1023, -90.7026) ccw construction
  arc A283 (-5.531, -93.5681) -> (-4.2799, -93.6336) centre (0, 0) ccw construction
  arc A284 (-6.3834, -91.8588) -> (-5.531, -93.5681) centre (-2.4177, -90.9481) ccw construction
  line L92 (-6.3834, -91.8588) -> (-6.5535, -91.1184) construction
  arc A285 (-6.5535, -91.1184) -> (-7.2762, -89.2805) centre (-13.0394, -92.6079) ccw construction
  arc A286 (-7.2762, -89.2805) -> (-11.4453, -88.8423) centre (-9.5199, -90.5759) ccw construction
  arc A287 (-11.4453, -88.8423) -> (-12.5343, -90.4898) centre (-6.4998, -93.2952) ccw construction
  line L93 (-12.5343, -90.4898) -> (-12.8546, -91.1787) construction
  arc A288 (-14.0438, -92.6733) -> (-12.8546, -91.1787) centre (-16.5444, -89.4633) ccw construction
  arc A289 (-15.2812, -92.4774) -> (-14.0438, -92.6733) centre (0, 0) ccw construction
  arc A290 (-15.9503, -90.6884) -> (-15.2812, -92.4774) centre (-11.9111, -90.1972) ccw construction
  line L94 (-15.9503, -90.6884) -> (-16.042, -89.9343) construction
  arc A291 (-16.042, -89.9343) -> (-16.5687, -88.0308) centre (-22.6482, -90.7376) ccw construction
  arc A292 (-16.5687, -88.0308) -> (-20.6691, -87.1593) centre (-18.9355, -89.0846) ccw construction
  arc A293 (-20.6691, -87.1593) -> (-21.9244, -88.6839) centre (-16.2162, -92.1048) ccw construction
  line L95 (-21.9244, -88.6839) -> (-22.3149, -89.3355) construction
  arc A294 (-23.6539, -90.6977) -> (-22.3149, -89.3355) centre (-25.8052, -87.2439) ccw construction
  arc A295 (-24.864, -90.3734) -> (-23.6539, -90.6977) centre (0, 0) ccw construction
  arc A296 (-25.3425, -88.5243) -> (-24.864, -90.3734) centre (-21.274, -88.458) ccw construction
  line L96 (-25.3425, -88.5243) -> (-25.3549, -87.7647) construction
  arc A297 (-25.3549, -87.7647) -> (-25.6797, -85.8167) centre (-32.0088, -87.8731) ccw construction
  arc A298 (-25.6797, -85.8167) -> (-29.6665, -84.5213) centre (-28.1437, -86.6173) ccw construction
  arc A299 (-29.6665, -84.5213) -> (-31.0743, -85.9064) centre (-25.7549, -89.9051) ccw construction
  line L97 (-31.0743, -85.9064) -> (-31.5308, -86.5136) construction
  arc A300 (-33.0048, -87.7283) -> (-31.5308, -86.5136) centre (-34.7833, -84.0686) ccw construction
  arc A301 (-34.1744, -87.2794) -> (-33.0048, -87.7283) centre (0, 0) ccw construction
  arc A302 (-34.457, -85.3903) -> (-34.1744, -87.2794) centre (-30.4038, -85.7497) ccw construction
  line L98 (-34.457, -85.3903) -> (-34.3899, -84.6337) construction
  arc A303 (-34.3899, -84.6337) -> (-34.5093, -82.6623) centre (-41.0187, -84.0459) ccw construction
  arc A304 (-34.5093, -82.6623) -> (-38.3389, -80.9573) centre (-37.0435, -83.201) ccw construction
  arc A305 (-38.3389, -80.9573) -> (-39.8838, -82.1876) centre (-35.0115, -86.7205) ccw construction
  line L99 (-39.8838, -82.1876) -> (-40.4012, -82.7438) construction
  arc A306 (-41.9941, -83.7978) -> (-40.4012, -82.7438) centre (-43.3803, -79.9722) ccw construction
  arc A307 (-43.1103, -83.2291) -> (-41.9941, -83.7978) centre (0, 0) ccw construction
  arc A308 (-43.1939, -81.3208) -> (-43.1103, -83.2291) centre (-39.2006, -82.1019) ccw construction
  line L100 (-43.1939, -81.3208) -> (-43.0481, -80.5753) construction
  arc A309 (-43.0481, -80.5753) -> (-42.9608, -78.6023) centre (-49.5792, -79.2979) ccw construction
  arc A310 (-42.9608, -78.6023) -> (-46.5912, -76.5063) centre (-45.5374, -78.8731) ccw construction
  arc A311 (-46.5912, -76.5063) -> (-48.2562, -77.5684) centre (-43.8844, -82.5858) ccw construction
  line L101 (-48.2562, -77.5684) -> (-48.829, -78.0674) construction
  arc A312 (-50.5233, -78.9492) -> (-48.829, -78.0674) centre (-51.502, -74.9996) ccw construction
  arc A313 (-51.574, -78.2669) -> (-50.5233, -78.9492) centre (0, 0) ccw construction
  arc A314 (-51.4576, -76.3604) -> (-51.574, -78.2669) centre (-47.5678, -77.5545) ccw construction
  line L102 (-51.4576, -76.3604) -> (-51.2347, -75.6342) construction
  arc A315 (-51.2347, -75.6342) -> (-50.9416, -73.6811) centre (-57.5964, -73.6811) ccw construction
  arc A316 (-50.9416, -73.6811) -> (-54.333, -71.2171) centre (-53.5324, -73.6811) ccw construction
  arc A317 (-54.333, -71.2171) -> (-56.1, -72.0993) centre (-52.2766, -77.5462) ccw construction
  line L103 (-56.1, -72.0993) -> (-56.7217, -72.5358) construction
  arc A318 (-58.499, -73.2356) -> (-56.7217, -72.5358) centre (-59.0595, -69.2054) ccw construction
  arc A319 (-59.4726, -72.4472) -> (-58.499, -73.2356) centre (0, 0) ccw construction
  arc A320 (-59.1576, -70.5633) -> (-59.4726, -72.4472) centre (-55.4139, -72.1575) ccw construction
  line L104 (-59.1576, -70.5633) -> (-58.8599, -69.8643) construction
  arc A321 (-58.8599, -69.8643) -> (-58.3643, -67.9526) centre (-64.9827, -67.257) ccw construction
  arc A322 (-58.3643, -67.9526) -> (-61.4796, -65.1476) centre (-60.941, -67.6818) ccw construction
  arc A323 (-61.4796, -65.1476) -> (-63.3291, -65.8403) centre (-60.096, -71.657) ccw construction
  line L105 (-63.3291, -65.8403) -> (-63.9931, -66.2094) construction
  arc A324 (-65.8337, -66.7196) -> (-63.9931, -66.2094) centre (-65.9699, -62.6528) ccw construction
  arc A325 (-66.7196, -65.8337) -> (-65.8337, -66.7196) centre (0, 0) ccw construction
  arc A326 (-66.2094, -63.9931) -> (-66.7196, -65.8337) centre (-62.6528, -65.9699) ccw construction
  line L106 (-66.2094, -63.9931) -> (-65.8403, -63.3291) construction
  arc A327 (-65.8403, -63.3291) -> (-65.1476, -61.4796) centre (-71.657, -60.096) ccw construction
  arc A328 (-65.1476, -61.4796) -> (-67.9526, -58.3643) centre (-67.6818, -60.9409) ccw construction
  arc A329 (-67.9526, -58.3643) -> (-69.8643, -58.8599) centre (-67.257, -64.9827) ccw construction
  line L107 (-69.8643, -58.8599) -> (-70.5633, -59.1576) construction
  arc A330 (-72.4472, -59.4726) -> (-70.5633, -59.1576) centre (-72.1575, -55.4139) ccw construction
  arc A331 (-73.2356, -58.499) -> (-72.4472, -59.4726) centre (0, 0) ccw construction
  arc A332 (-72.5358, -56.7217) -> (-73.2356, -58.499) centre (-69.2054, -59.0595) ccw construction
  line L108 (-72.5358, -56.7217) -> (-72.0993, -56.1) construction
  arc A333 (-72.0993, -56.1) -> (-71.2171, -54.333) centre (-77.5462, -52.2766) ccw construction
  arc A334 (-71.2171, -54.333) -> (-73.6811, -50.9416) centre (-73.6811, -53.5324) ccw construction
  arc A335 (-73.6811, -50.9416) -> (-75.6342, -51.2347) centre (-73.6811, -57.5964) ccw construction
  line L109 (-75.6342, -51.2347) -> (-76.3604, -51.4576) construction
  arc A336 (-78.2669, -51.574) -> (-76.3604, -51.4576) centre (-77.5546, -47.5678) ccw construction
  arc A337 (-78.9492, -50.5233) -> (-78.2669, -51.574) centre (0, 0) ccw construction
  arc A338 (-78.0675, -48.829) -> (-78.9492, -50.5233) centre (-74.9996, -51.502) ccw construction
  line L110 (-78.0675, -48.829) -> (-77.5684, -48.2562) construction
  arc A339 (-77.5684, -48.2562) -> (-76.5063, -46.5912) centre (-82.5858, -43.8844) ccw construction
  arc A340 (-76.5063, -46.5912) -> (-78.6023, -42.9608) centre (-78.8731, -45.5374) ccw construction
  arc A341 (-78.6023, -42.9608) -> (-80.5753, -43.0481) centre (-79.2979, -49.5791) ccw construction
  line L111 (-80.5753, -43.0481) -> (-81.3208, -43.1939) construction
  arc A342 (-83.2291, -43.1103) -> (-81.3208, -43.1939) centre (-82.1019, -39.2006) ccw construction
  arc A343 (-83.7978, -41.9941) -> (-83.2291, -43.1103) centre (0, 0) ccw construction
  arc A344 (-82.7438, -40.4012) -> (-83.7978, -41.9941) centre (-79.9722, -43.3803) ccw construction
  line L112 (-82.7438, -40.4012) -> (-82.1876, -39.8838) construction
  arc A345 (-82.1876, -39.8838) -> (-80.9573, -38.3389) centre (-86.7205, -35.0115) ccw construction
  arc A346 (-80.9573, -38.3389) -> (-82.6623, -34.5093) centre (-83.201, -37.0435) ccw construction
  arc A347 (-82.6623, -34.5093) -> (-84.6337, -34.3899) centre (-84.0459, -41.0187) ccw construction
  line L113 (-84.6337, -34.3899) -> (-85.3904, -34.4569) construction
  arc A348 (-87.2794, -34.1744) -> (-85.3904, -34.4569) centre (-85.7497, -30.4038) ccw construction
  arc A349 (-87.7283, -33.0048) -> (-87.2794, -34.1744) centre (0, 0) ccw construction
  arc A350 (-86.5136, -31.5308) -> (-87.7283, -33.0048) centre (-84.0686, -34.7833) ccw construction
  line L114 (-86.5136, -31.5308) -> (-85.9064, -31.0743) construction
  arc A351 (-85.9064, -31.0743) -> (-84.5213, -29.6665) centre (-89.9052, -25.7549) ccw construction
  arc A352 (-84.5213, -29.6665) -> (-85.8167, -25.6797) centre (-86.6173, -28.1437) ccw construction
  arc A353 (-85.8167, -25.6797) -> (-87.7647, -25.3548) centre (-87.8732, -32.0088) ccw construction
  line L115 (-87.7647, -25.3548) -> (-88.5243, -25.3425) construction
  arc A354 (-90.3734, -24.864) -> (-88.5243, -25.3425) centre (-88.458, -21.274) ccw construction
  arc A355 (-90.6977, -23.6539) -> (-90.3734, -24.864) centre (0, 0) ccw construction
  arc A356 (-89.3355, -22.3149) -> (-90.6977, -23.6539) centre (-87.2439, -25.8052) ccw construction
  line L116 (-89.3355, -22.3149) -> (-88.6839, -21.9244) construction
  arc A357 (-88.6839, -21.9244) -> (-87.1593, -20.6691) centre (-92.1048, -16.2162) ccw construction
  arc A358 (-87.1593, -20.6691) -> (-88.0308, -16.5687) centre (-89.0846, -18.9355) ccw construction
  arc A359 (-88.0308, -16.5687) -> (-89.9343, -16.042) centre (-90.7376, -22.6482) ccw construction
  line L117 (-89.9343, -16.042) -> (-90.6884, -15.9503) construction
  arc A360 (-92.4774, -15.2812) -> (-90.6884, -15.9503) centre (-90.1972, -11.9111) ccw construction
  arc A361 (-92.6733, -14.0438) -> (-92.4774, -15.2812) centre (0, 0) ccw construction
  arc A362 (-91.1787, -12.8546) -> (-92.6733, -14.0438) centre (-89.4633, -16.5443) ccw construction
  line L118 (-91.1787, -12.8546) -> (-90.4898, -12.5343) construction
  arc A363 (-90.4898, -12.5343) -> (-88.8423, -11.4453) centre (-93.2953, -6.4998) ccw construction
  arc A364 (-88.8423, -11.4453) -> (-89.2805, -7.2762) centre (-90.5759, -9.5199) ccw construction
  arc A365 (-89.2805, -7.2762) -> (-91.1184, -6.5535) centre (-92.6079, -13.0394) ccw construction
  line L119 (-91.1184, -6.5535) -> (-91.8588, -6.3834) construction
  arc A366 (-93.5681, -5.531) -> (-91.8588, -6.3834) centre (-90.9481, -2.4177) ccw construction
  line L120 (-5.251, 19.7934) -> (-6.1577, 23.1772) construction
  arc A367 (-6.1577, 23.1772) -> (-7.4205, 23.8733) centre (-7.1237, 22.9184) ccw construction
  arc A368 (-7.4205, 23.8733) -> (-16.9452, 18.3809) centre (0, 0) ccw construction
  arc A369 (-16.9452, 18.3809) -> (-16.9745, 16.9386) centre (-16.2674, 17.6457) ccw construction
  line L121 (-16.9745, 16.9386) -> (-14.4973, 14.4613) construction
  arc A370 (-14.4973, 14.4613) -> (-13.1175, 14.4285) centre (-13.7902, 15.1684) ccw construction
  arc A371 (-5.9137, 18.5817) -> (-13.1175, 14.4285) centre (0, 0) ccw construction
  arc A372 (-5.9137, 18.5817) -> (-5.251, 19.7934) centre (-6.217, 19.5346) ccw construction
  line L122 (-19.7671, 5.3492) -> (-23.1509, 6.2559) construction
  arc A373 (-23.1509, 6.2559) -> (-24.3852, 5.5104) centre (-23.4098, 5.2899) ccw construction
  arc A374 (-24.3852, 5.5104) -> (-24.391, -5.4845) centre (0, 0) ccw construction
  arc A375 (-24.391, -5.4845) -> (-23.1565, -6.2311) centre (-23.4153, -5.2651) ccw construction
  line L123 (-23.1565, -6.2311) -> (-19.7725, -5.3243) construction
  arc A376 (-19.7725, -5.3243) -> (-19.0542, -4.1458) centre (-20.0313, -4.3584) ccw construction
  arc A377 (-19.049, 4.1694) -> (-19.0542, -4.1458) centre (0, 0) ccw construction
  arc A378 (-19.049, 4.1694) -> (-19.7671, 5.3492) centre (-20.0259, 4.3832) ccw construction
  arc A379 (-13.1353, -14.4122) -> (-5.9367, -18.5743) centre (0, 0) ccw construction
  arc A380 (-13.1353, -14.4122) -> (-14.5161, -14.4442) centre (-13.809, -15.1513) ccw construction
  line L124 (-14.5161, -14.4442) -> (-16.9932, -16.9214) construction
  arc A381 (-16.9932, -16.9214) -> (-16.9647, -18.363) centre (-16.2861, -17.6285) ccw construction
  arc A382 (-16.9647, -18.363) -> (-7.4458, -23.8655) centre (0, 0) ccw construction
  arc A383 (-7.4458, -23.8655) -> (-6.182, -23.1697) centre (-7.1479, -22.9109) ccw construction
  line L125 (-6.182, -23.1697) -> (-5.2753, -19.7857) construction
  arc A384 (-5.2753, -19.7857) -> (-5.9367, -18.5743) centre (-6.2412, -19.5268) ccw construction
  line L126 (16.9745, -16.9386) -> (14.4973, -14.4613) construction
  arc A385 (14.4973, -14.4613) -> (13.1175, -14.4285) centre (13.7902, -15.1684) ccw construction
  arc A386 (5.9137, -18.5817) -> (13.1175, -14.4285) centre (0, 0) ccw construction
  arc A387 (5.9137, -18.5817) -> (5.251, -19.7934) centre (6.217, -19.5346) ccw construction
  line L127 (5.251, -19.7934) -> (6.1577, -23.1772) construction
  arc A388 (6.1577, -23.1772) -> (7.4205, -23.8733) centre (7.1237, -22.9184) ccw construction
  arc A389 (7.4205, -23.8733) -> (16.9452, -18.3809) centre (0, 0) ccw construction
  arc A390 (16.9452, -18.3809) -> (16.9745, -16.9386) centre (16.2674, -17.6457) ccw construction
  arc A391 (24.3852, -5.5104) -> (24.391, 5.4845) centre (0, 0) ccw construction
  arc A392 (24.391, 5.4845) -> (23.1565, 6.2311) centre (23.4153, 5.2651) ccw construction
  line L128 (23.1565, 6.2311) -> (19.7725, 5.3243) construction
  arc A393 (19.7725, 5.3243) -> (19.0542, 4.1458) centre (20.0313, 4.3584) ccw construction
  arc A394 (19.049, -4.1694) -> (19.0542, 4.1458) centre (0, 0) ccw construction
  arc A395 (19.049, -4.1694) -> (19.7671, -5.3492) centre (20.0259, -4.3832) ccw construction
  line L129 (19.7671, -5.3492) -> (23.1509, -6.2559) construction
  arc A396 (23.1509, -6.2559) -> (24.3852, -5.5104) centre (23.4098, -5.2899) ccw construction
  line L130 (14.5161, 14.4442) -> (16.9932, 16.9214) construction
  arc A397 (16.9932, 16.9214) -> (16.9647, 18.363) centre (16.2861, 17.6285) ccw construction
  arc A398 (16.9647, 18.363) -> (7.4458, 23.8655) centre (0, 0) ccw construction
  arc A399 (7.4458, 23.8655) -> (6.182, 23.1697) centre (7.1479, 22.9109) ccw construction
  line L131 (6.182, 23.1697) -> (5.2753, 19.7857) construction
  arc A400 (5.2753, 19.7857) -> (5.9367, 18.5743) centre (6.2412, 19.5268) ccw construction
  arc A401 (13.1353, 14.4122) -> (5.9367, 18.5743) centre (0, 0) ccw construction
  arc A402 (13.1353, 14.4122) -> (14.5161, 14.4442) centre (13.809, 15.1513) ccw construction
  line L132 (101.6, -101.6) -> (-101.6, -101.6)
  line L133 (-101.6, -101.6) -> (-101.6, 101.6) construction
  line L134 (-101.6, 101.6) -> (101.6, 101.6) construction
  line L135 (101.6, 101.6) -> (101.6, -101.6)
  line L136 (101.6, -101.6) -> (-101.6, 101.6) construction
  line L137 (-101.6, -101.6) -> (101.6, 101.6) construction
  line L138 (-101.6, -101.6) -> (-101.6, 101.6) projected
  line L139 (-101.6, 101.6) -> (101.6, 101.6) projected
  arc A403 (-71.3122, 54.3021) -> (-72.1812, 56.0425) centre (-77.5462, 52.2766) ccw
  arc A404 (-73.6811, 51.0416) -> (-71.3122, 54.3021) centre (-73.6811, 53.5324) ccw
  arc A405 (-75.6048, 51.3303) -> (-73.6811, 51.0416) centre (-73.6811, 57.5964) ccw
  line L140 (-75.6048, 51.3303) -> (-76.331, 51.5532)
  arc A406 (-76.331, 51.5532) -> (-78.3269, 51.6647) centre (-77.5546, 47.5678) ccw
  arc A407 (-78.3269, 51.6647) -> (-79.0564, 50.5412) centre (0, 0) ccw
  arc A408 (-79.0564, 50.5412) -> (-78.1428, 48.7633) centre (-74.9996, 51.502) ccw
  line L141 (-78.1428, 48.7633) -> (-77.6438, 48.1905)
  arc A409 (-76.5977, 46.5505) -> (-77.6438, 48.1905) centre (-82.5858, 43.8844) ccw
  arc A410 (-78.6128, 43.0603) -> (-76.5977, 46.5505) centre (-78.8731, 45.5374) ccw
  arc A411 (-80.5561, 43.1462) -> (-78.6128, 43.0603) centre (-79.2979, 49.5791) ccw
  line L142 (-80.5561, 43.1462) -> (-81.3016, 43.2921)
  arc A412 (-81.3016, 43.2921) -> (-83.2982, 43.1942) centre (-82.1019, 39.2006) ccw
  arc A413 (-83.2982, 43.1942) -> (-83.9063, 42.0007) centre (0, 0) ccw
  arc A414 (-83.9063, 42.0007) -> (-82.8119, 40.328) centre (-79.9722, 43.3803) ccw
  line L143 (-82.8119, 40.328) -> (-82.2557, 39.8105)
  arc A415 (-81.0439, 38.2889) -> (-82.2557, 39.8105) centre (-86.7205, 35.0115) ccw
  arc A416 (-82.6831, 34.6071) -> (-81.0439, 38.2889) centre (-83.201, 37.0435) ccw
  arc A417 (-84.6248, 34.4895) -> (-82.6831, 34.6071) centre (-84.0459, 41.0187) ccw
  line L144 (-84.6248, 34.4895) -> (-85.3815, 34.5566)
  arc A418 (-85.3815, 34.5566) -> (-87.3569, 34.2506) centre (-85.7497, 30.4038) ccw
  arc A419 (-87.3569, 34.2506) -> (-87.837, 33) centre (0, 0) ccw